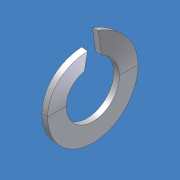
# Autodesk Inventor part: Washer-Spring5
Saved by Autodesk Inventor 2014 SP1 (Build 180222100, 222)
## iProperties
Category: PARTsolutions
Created: 2015-02-04
Part Number: Washer-Spring5
Catalog Web Link: www.cadenas.de
Description: hcbstspringwasher - Washer Assembled Hexagon Socket Head Cap Screws
Document SubType Name: Modeling
Designer: PARTsolutions
Material: Generic
Density: 1 g/cm^3
Appearance: RGB(192,192,192)
NB: Washer-Spring5
NN: hcbstspringwasher
NT: Washer Assembled Hexagon Socket Head Cap Screws
NBSYN: $PN.
LINA: Washer-Spring5
PN: Washer-Spring5
M: 5
M1: 5.000
MP: 5x0.8
P: 0.800
C: 8.5
D: 10.0
AA: 5.4
KT: DUMMY
SUPPLIER: Misumi
ARTICLENO: Washer-Spring5
BOMINFO: Washer-Spring5
CREATOR: CADENAS GmbH
PSOL_IDENT_0: {\\10.0.0.236\data_v8\23d-libs\misumi\metric\38_al_extrusions_blackets\nuts\hcbst_wash_s.prj},181 {V
PSOL_IDENT_1: TYP=3D},{NB=Washer-Spring5},{LINA=Washer-Spring5},{NN=hcbstspringwasher},{DATE=19.11.2014 02:34:01},
PSOL_IDENT_2: {GEOMDATE=19.11.2007 11:50:00},{VERSION=},{LINEID=40},{LINESUBID=-1},{WBVAR=}  {NB=Washer-Spring5},{
PSOL_IDENT_3: LINA=Washer-Spring5},{KT=DUMMY},{PN=Washer-Spring5},{M=5},{M1=5.000},{MP=5x0.8},{P=0.8},{C=8.5},{D=1
PSOL_IDENT_4: 0.0},{AA=5.4}
Title: Washer-Spring5
Author: Cadenas PARTsolutions
Comments: Washer Assembled Hexagon Socket Head Cap Screws
Autodesk Inventor part; units mm, degrees
sketch "Sketch_1" plane through (0, 0, 0) normal (0, 0, 1) x (1, 0, 0)
  line L0 (0.27, 0) -> (-0.27, 0)
  line L1 (-0.27, 0) -> (-0.27, 4.25)
  line L2 (-0.27, 4.25) -> (0.27, 4.25)
  line L3 (0.27, 4.25) -> (0.27, 0)
  line L4 (0.27, 0) -> (-0.27, 0)
  constraints: 10 end point
revolve "Revolution1" add sketch "Sketch_1" angle 180 about axis through (0.27, 0, 0) along (-1, 0, 0)
sketch "Sketch_2" plane through (0, 0, 0) normal (0, 0, 1) x (1, 0, 0)
  line L0 (0.27, -0.0476) -> (-0.27, 0.0476)
  line L1 (-0.27, 0.0476) -> (-0.27, 4.25)
  line L2 (-0.27, 4.25) -> (0.27, 4.25)
  line L3 (0.27, 4.25) -> (0.27, -0.0476)
  line L4 (0.27, -0.0476) -> (-0.27, 0.0476)
  constraints: 10 end point
revolve "Revolution2" add sketch "Sketch_2" angle 90 about axis through (0.27, -0.0476, 0) along (0.9848078, -0.1736482, 0)
sketch "Sketch_3" plane through (0, 0, 0) normal (0, 0, 1) x (1, 0, 0)
  line L0 (-0.27, 0.0476) -> (0.27, -0.0476)
  line L1 (0.27, -0.0476) -> (0.27, -4.25)
  line L2 (0.27, -4.25) -> (-0.27, -4.25)
  line L3 (-0.27, -4.25) -> (-0.27, 0.0476)
  line L4 (-0.27, 0.0476) -> (0.27, -0.0476)
  constraints: 10 end point
revolve "Revolution3" add sketch "Sketch_3" angle 90 about axis through (-0.27, 0.0476, 0) along (-0.9848078, 0.1736482, 0)
sketch "Sketch_4" plane through (0, 0, 0) normal (1, 0, 0) x (0, 1, 0)
  line L0 (-1.0625, 4.25) -> (-1.0625, 2.263)
  arc A0 (-1.0625, 2.263) -> (1.0625, 2.263) centre (0, 0) ccw
  line L1 (1.0625, 2.263) -> (1.0625, 4.25)
  line L2 (1.0625, 4.25) -> (-1.0625, 4.25)
  constraints: 6 end point, 2 point on circle, 1 centre point
extrude "Extrusion1" cut sketch "Sketch_4" along normal mid plane 17
ref_plane "spring_washer_to_bolt_XY" through (0, 0, 0) normal (1, 0, 0) x (0, 0, -1)
ref_plane "spring_washer_to_bolt_YZ" through (0, 0, 0) normal (0, 0, -1) x (0, 1, 0)
ref_plane "spring_washer_to_bolt_ZX" through (0, 0, 0) normal (0, 1, 0) x (1, 0, 0)
body "Solid1"
